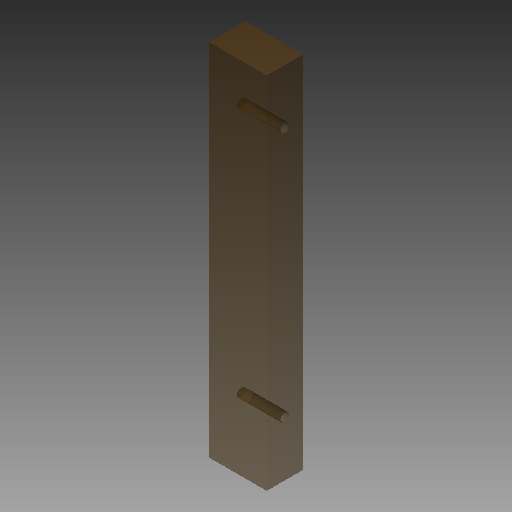
# Autodesk Inventor part: Abstreifer
Saved by Autodesk Inventor 2018 (Build 220112000, 112)
## iProperties
Created: 2013-02-21
Part Number: Abstreifer
Material: Polycarbonate, Smoke
Document SubType Name: Modeling
Designer: Neef
Mass: 18.8892 g
Surface Area: 54.462 cm^2
Volume: 15.741 cm^3
Density: 1.2 g/cm^3
Appearance: Polycarbonate - Smoked
Author: Neef
Autodesk Inventor part; units mm, degrees
ref_plane "YZ Plane" through (0, 0, 0) normal (1, 0, 0) x (0, 1, 0)
ref_plane "XZ Plane" through (0, 0, 0) normal (0, 1, 0) x (-1, 0, 0)
ref_plane "XY Plane" through (0, 0, 0) normal (0, 0, 1) x (1, 0, 0)
sketch "Skizze1" plane through (0, 0, 0) normal (0, 0, 1) x (1, 0, 0)
  line L0 (-7.95, 5) -> (7.95, 5)
  line L1 (7.95, 5) -> (7.95, -5)
  line L2 (7.95, -5) -> (-7.95, -5)
  line L3 (-7.95, -5) -> (-7.95, 5)
  line L4 (0, 7) -> (0, -7) projected
  line L5 (-11.13, 0) -> (11.13, 0) projected
  point P0 (0, 0)
  point P1 (0, 5)
  point P2 (-7.95, 0)
  dimension "d0" = 15.9
  dimension "d1" = 10
  constraints: 8 end point, 2 midpoint, 2 parallel, 2 point on line, 1 horizontal, 1 perpendicular
  measures "d0" distance of L0.start L0.end
  measures "d1" distance of L2.end L0.start
extrude "Extrusion1" add sketch "Skizze1" along normal blind 99
sketch "Skizze2" plane through (7.95, -5, 0) normal (1, 0, 0) x (0, 0, -1)
  line L0 (-99, 10) -> (-99, 0) projected
  line L1 (0, 0) -> (0, 10) projected
  line L2 (0, 10) -> (-99, 10) projected
  point P0 (0, 5)
  point P1 (-84, 5)
  point P2 (-15, 5)
  dimension "d4" = 15
  dimension "d5" = 15
  dimension "d6" = 5
  dimension "d7" = 5
  measures "d4" distance from line of L0 point (-84, 5)
  measures "d5" distance from line of L1 point (-15, 5)
  measures "d6" distance from line of L2 point (-84, 5)
  measures "d7" distance from line of L2 point (-15, 5)
hole "Bohrung1" at (7.95, 0, 84) at (7.95, 0, 15) direction (-1, 0, 0) diameter 2.459 depth 12 tip angle 118 thread size "M3x0.5" class "6H" standard "ISO Metric profile"
